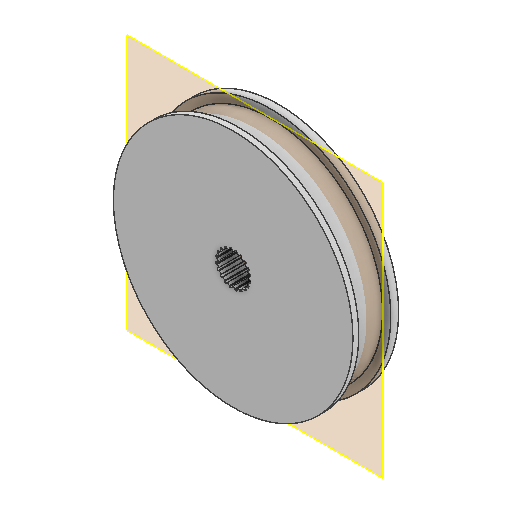
# Autodesk Inventor part: Diff Large Pulley
Saved by Autodesk Inventor 2025.2 (Build 292293000, 293)
## iProperties
Created: 2025-02-20
Part Number: Diff Large Pulley
Material: Generic
Document SubType Name: Modeling
Designer: Jakeg
Density: 1 g/cm^3
Appearance: Default
Author: Jakeg
Autodesk Inventor part; units mm, degrees
ref_plane "YZ Plane" through (0, 0, 0) normal (1, 0, 0) x (0, 1, 0)
ref_plane "XZ Plane" through (0, 0, 0) normal (0, 1, 0) x (-1, 0, 0)
ref_plane "XY Plane" through (0, 0, 0) normal (0, 0, 1) x (1, 0, 0)
sketch "Sketch1" plane through (0, 0, 0) normal (0, 0, 1) x (1, 0, 0)
  circle A0 centre (0, 0) radius 41.14
  dimension "d0" = 82.28
  constraints: 1 centre point, 1 coincident
  measures "d0" diameter of A0
extrude "Extrusion1" add sketch "Sketch1" along normal blind 15.7
ref_plane "Work Plane1" through (0, 0, 8.2) normal (0, 0, 1) x (1, 0, 0)
sketch "Sketch2" plane through (0, 0, 8.2) normal (0, 0, 1) x (1, 0, 0)
  circle A0 centre (0, 0) radius 38.3
  circle A1 centre (0, 0) radius 41.14
  dimension "d4" = 76.6
  constraints: 2 centre point, 2 coincident
  measures "d4" diameter of A0
extrude "Extrusion2" cut sketch "Sketch2" along normal mid plane 11
sketch "Sketch3" plane through (0, 0, 15.7) normal (0, 0, 1) x (1, 0, 0)
  circle A0 centre (0, 0) radius 6
  circle A1 centre (0, 20.32) radius 3.175
  circle A2 centre (0, -20.32) radius 3.175
  dimension "d7" = 12
  dimension "d13" = 6.35
  dimension "d14" = 20.32
  dimension "d15" = 6.35
  dimension "d16" = 20.32
  constraints: 3 centre point, 1 coincident
  measures "d7" diameter of A0
  measures "d13" diameter of A1
  measures "d14" distance of point (0, 0) A1.centre
  measures "d15" diameter of A2
  measures "d16" distance of point (0, 0) A2.centre
extrude "Extrusion3" cut sketch "Sketch3" against normal through all contours A0
sketch "Sketch5" plane through (0, 0, 15.7) normal (0, 0, 1) x (1, 0, 0)
  circle A0 centre (0, 0) radius 6 projected
  arc A1 (-1.2778, -5.5469) -> (-2.2267, -5.2386) centre (-1.8274, -5.6241) ccw
  arc A2 (-1.2783, -5.8289) -> (-1.2778, -5.5469) centre (-2.2681, -5.6859) ccw
  arc A3 (-1.2783, -5.8289) -> (-1.1583, -5.9977) centre (-1.1299, -5.8504) ccw
  arc A4 (-1.1583, -5.9977) -> (-0.7518, -6.0621) centre (0, 0) ccw
  arc A5 (-0.7518, -6.0621) -> (-0.5855, -5.9387) centre (-0.7333, -5.9132) ccw
  arc A6 (-0.4989, -5.6703) -> (-0.5855, -5.9387) centre (0.4, -6.1085) ccw
  arc A7 (0.4989, -5.6703) -> (-0.4989, -5.6703) centre (0, -5.9135) ccw
  arc A8 (0.5855, -5.9387) -> (0.4989, -5.6703) centre (-0.4, -6.1085) ccw
  arc A9 (0.5855, -5.9387) -> (0.7518, -6.0621) centre (0.7333, -5.9132) ccw
  arc A10 (0.7518, -6.0621) -> (1.1583, -5.9977) centre (0, 0) ccw
  arc A11 (1.1583, -5.9977) -> (1.2783, -5.8289) centre (1.1299, -5.8504) ccw
  arc A12 (1.2778, -5.5469) -> (1.2783, -5.8289) centre (2.2681, -5.6859) ccw
  arc A13 (2.2267, -5.2386) -> (1.2778, -5.5469) centre (1.8274, -5.6241) ccw
  arc A14 (2.392, -5.4671) -> (2.2267, -5.2386) centre (1.5072, -5.9331) ccw
  arc A15 (2.392, -5.4671) -> (2.5882, -5.5331) centre (2.5247, -5.3972) ccw
  arc A16 (2.5882, -5.5331) -> (2.955, -5.3462) centre (0, 0) ccw
  arc A17 (2.955, -5.3462) -> (3.017, -5.1486) centre (2.8824, -5.2149) ccw
  arc A18 (2.9293, -4.8806) -> (3.017, -5.1486) centre (3.9141, -4.7068) ccw
  arc A19 (3.7365, -4.2941) -> (2.9293, -4.8806) centre (3.4759, -4.7841) ccw
  arc A20 (3.9643, -4.4604) -> (3.7365, -4.2941) centre (3.2669, -5.177) ccw
  arc A21 (3.9643, -4.4604) -> (4.1714, -4.4624) centre (4.0689, -4.3529) ccw
  arc A22 (4.1714, -4.4624) -> (4.4624, -4.1714) centre (0, 0) ccw
  arc A23 (4.4624, -4.1714) -> (4.4604, -3.9643) centre (4.3529, -4.0689) ccw
  arc A24 (4.2941, -3.7365) -> (4.4604, -3.9643) centre (5.177, -3.2669) ccw
  arc A25 (4.8806, -2.9293) -> (4.2941, -3.7365) centre (4.7841, -3.4759) ccw
  arc A26 (5.1486, -3.017) -> (4.8806, -2.9293) centre (4.7068, -3.9141) ccw
  arc A27 (5.1486, -3.017) -> (5.3462, -2.955) centre (5.2149, -2.8824) ccw
  arc A28 (5.3462, -2.955) -> (5.5331, -2.5882) centre (0, 0) ccw
  arc A29 (5.5331, -2.5882) -> (5.4671, -2.392) centre (5.3972, -2.5247) ccw
  arc A30 (5.2386, -2.2267) -> (5.4671, -2.392) centre (5.9331, -1.5072) ccw
  arc A31 (5.5469, -1.2778) -> (5.2386, -2.2267) centre (5.6241, -1.8274) ccw
  arc A32 (5.8289, -1.2783) -> (5.5469, -1.2778) centre (5.6859, -2.2681) ccw
  arc A33 (5.8289, -1.2783) -> (5.9977, -1.1583) centre (5.8504, -1.1299) ccw
  arc A34 (5.9977, -1.1583) -> (6.0621, -0.7518) centre (0, 0) ccw
  arc A35 (6.0621, -0.7518) -> (5.9387, -0.5855) centre (5.9132, -0.7333) ccw
  arc A36 (5.6703, -0.4989) -> (5.9387, -0.5855) centre (6.1085, 0.4) ccw
  arc A37 (5.6703, 0.4989) -> (5.6703, -0.4989) centre (5.9135, 0) ccw
  arc A38 (5.9387, 0.5855) -> (5.6703, 0.4989) centre (6.1085, -0.4) ccw
  arc A39 (5.9387, 0.5855) -> (6.0621, 0.7518) centre (5.9132, 0.7333) ccw
  arc A40 (6.0621, 0.7518) -> (5.9977, 1.1583) centre (0, 0) ccw
  arc A41 (5.9977, 1.1583) -> (5.8289, 1.2783) centre (5.8504, 1.1299) ccw
  arc A42 (5.5469, 1.2778) -> (5.8289, 1.2783) centre (5.6859, 2.2681) ccw
  arc A43 (5.2386, 2.2267) -> (5.5469, 1.2778) centre (5.6241, 1.8274) ccw
  arc A44 (5.4671, 2.392) -> (5.2386, 2.2267) centre (5.9331, 1.5072) ccw
  arc A45 (5.4671, 2.392) -> (5.5331, 2.5882) centre (5.3972, 2.5247) ccw
  arc A46 (5.5331, 2.5882) -> (5.3462, 2.955) centre (0, 0) ccw
  arc A47 (5.3462, 2.955) -> (5.1486, 3.017) centre (5.2149, 2.8824) ccw
  arc A48 (4.8806, 2.9293) -> (5.1486, 3.017) centre (4.7068, 3.9141) ccw
  arc A49 (4.2941, 3.7365) -> (4.8806, 2.9293) centre (4.7841, 3.4759) ccw
  arc A50 (4.4604, 3.9643) -> (4.2941, 3.7365) centre (5.177, 3.2669) ccw
  arc A51 (4.4604, 3.9643) -> (4.4624, 4.1714) centre (4.3529, 4.0689) ccw
  arc A52 (4.4624, 4.1714) -> (4.1714, 4.4624) centre (0, 0) ccw
  arc A53 (4.1714, 4.4624) -> (3.9643, 4.4604) centre (4.0689, 4.3529) ccw
  arc A54 (3.7365, 4.2941) -> (3.9643, 4.4604) centre (3.2669, 5.177) ccw
  arc A55 (2.9293, 4.8806) -> (3.7365, 4.2941) centre (3.4759, 4.7841) ccw
  arc A56 (3.017, 5.1486) -> (2.9293, 4.8806) centre (3.9141, 4.7068) ccw
  arc A57 (3.017, 5.1486) -> (2.955, 5.3462) centre (2.8824, 5.2149) ccw
  arc A58 (2.955, 5.3462) -> (2.5882, 5.5331) centre (0, 0) ccw
  arc A59 (2.5882, 5.5331) -> (2.392, 5.4671) centre (2.5247, 5.3972) ccw
  arc A60 (2.2267, 5.2386) -> (2.392, 5.4671) centre (1.5072, 5.9331) ccw
  arc A61 (1.2778, 5.5469) -> (2.2267, 5.2386) centre (1.8274, 5.6241) ccw
  arc A62 (1.2783, 5.8289) -> (1.2778, 5.5469) centre (2.2681, 5.6859) ccw
  arc A63 (1.2783, 5.8289) -> (1.1583, 5.9977) centre (1.1299, 5.8504) ccw
  arc A64 (1.1583, 5.9977) -> (0.7518, 6.0621) centre (0, 0) ccw
  arc A65 (0.7518, 6.0621) -> (0.5855, 5.9387) centre (0.7333, 5.9132) ccw
  arc A66 (0.4989, 5.6703) -> (0.5855, 5.9387) centre (-0.4, 6.1085) ccw
  arc A67 (-0.4989, 5.6703) -> (0.4989, 5.6703) centre (0, 5.9135) ccw
  arc A68 (-0.5855, 5.9387) -> (-0.4989, 5.6703) centre (0.4, 6.1085) ccw
  arc A69 (-0.5855, 5.9387) -> (-0.7518, 6.0621) centre (-0.7333, 5.9132) ccw
  arc A70 (-0.7518, 6.0621) -> (-1.1583, 5.9977) centre (0, 0) ccw
  arc A71 (-1.1583, 5.9977) -> (-1.2783, 5.8289) centre (-1.1299, 5.8504) ccw
  arc A72 (-1.2778, 5.5469) -> (-1.2783, 5.8289) centre (-2.2681, 5.6859) ccw
  arc A73 (-2.2267, 5.2386) -> (-1.2778, 5.5469) centre (-1.8274, 5.6241) ccw
  arc A74 (-2.392, 5.4671) -> (-2.2267, 5.2386) centre (-1.5072, 5.9331) ccw
  arc A75 (-2.392, 5.4671) -> (-2.5882, 5.5331) centre (-2.5247, 5.3972) ccw
  arc A76 (-2.5882, 5.5331) -> (-2.955, 5.3462) centre (0, 0) ccw
  arc A77 (-2.955, 5.3462) -> (-3.017, 5.1486) centre (-2.8824, 5.2149) ccw
  arc A78 (-2.9293, 4.8806) -> (-3.017, 5.1486) centre (-3.9141, 4.7068) ccw
  arc A79 (-3.7365, 4.2941) -> (-2.9293, 4.8806) centre (-3.4759, 4.7841) ccw
  arc A80 (-3.9643, 4.4604) -> (-3.7365, 4.2941) centre (-3.2669, 5.177) ccw
  arc A81 (-3.9643, 4.4604) -> (-4.1714, 4.4624) centre (-4.0689, 4.3529) ccw
  arc A82 (-4.1714, 4.4624) -> (-4.4624, 4.1714) centre (0, 0) ccw
  arc A83 (-4.4624, 4.1714) -> (-4.4604, 3.9643) centre (-4.3529, 4.0689) ccw
  arc A84 (-4.2941, 3.7365) -> (-4.4604, 3.9643) centre (-5.177, 3.2669) ccw
  arc A85 (-4.8806, 2.9293) -> (-4.2941, 3.7365) centre (-4.7841, 3.4759) ccw
  arc A86 (-5.1486, 3.017) -> (-4.8806, 2.9293) centre (-4.7068, 3.9141) ccw
  arc A87 (-5.1486, 3.017) -> (-5.3462, 2.955) centre (-5.2149, 2.8824) ccw
  arc A88 (-5.3462, 2.955) -> (-5.5331, 2.5882) centre (0, 0) ccw
  arc A89 (-5.5331, 2.5882) -> (-5.4671, 2.392) centre (-5.3972, 2.5247) ccw
  arc A90 (-5.2386, 2.2267) -> (-5.4671, 2.392) centre (-5.9331, 1.5072) ccw
  arc A91 (-5.5469, 1.2778) -> (-5.2386, 2.2267) centre (-5.6241, 1.8274) ccw
  arc A92 (-5.8289, 1.2783) -> (-5.5469, 1.2778) centre (-5.6859, 2.2681) ccw
  arc A93 (-5.8289, 1.2783) -> (-5.9977, 1.1583) centre (-5.8504, 1.1299) ccw
  arc A94 (-5.9977, 1.1583) -> (-6.0621, 0.7518) centre (0, 0) ccw
  arc A95 (-6.0621, 0.7518) -> (-5.9387, 0.5855) centre (-5.9132, 0.7333) ccw
  arc A96 (-5.6703, 0.4989) -> (-5.9387, 0.5855) centre (-6.1085, -0.4) ccw
  arc A97 (-5.6703, -0.4989) -> (-5.6703, 0.4989) centre (-5.9135, 0) ccw
  arc A98 (-5.9387, -0.5855) -> (-5.6703, -0.4989) centre (-6.1085, 0.4) ccw
  arc A99 (-5.9387, -0.5855) -> (-6.0621, -0.7518) centre (-5.9132, -0.7333) ccw
  arc A100 (-6.0621, -0.7518) -> (-5.9977, -1.1583) centre (0, 0) ccw
  arc A101 (-5.9977, -1.1583) -> (-5.8289, -1.2783) centre (-5.8504, -1.1299) ccw
  arc A102 (-5.5469, -1.2778) -> (-5.8289, -1.2783) centre (-5.6859, -2.2681) ccw
  arc A103 (-5.2386, -2.2267) -> (-5.5469, -1.2778) centre (-5.6241, -1.8274) ccw
  arc A104 (-5.4671, -2.392) -> (-5.2386, -2.2267) centre (-5.9331, -1.5072) ccw
  arc A105 (-5.4671, -2.392) -> (-5.5331, -2.5882) centre (-5.3972, -2.5247) ccw
  arc A106 (-5.5331, -2.5882) -> (-5.3462, -2.955) centre (0, 0) ccw
  arc A107 (-5.3462, -2.955) -> (-5.1486, -3.017) centre (-5.2149, -2.8824) ccw
  arc A108 (-4.8806, -2.9293) -> (-5.1486, -3.017) centre (-4.7068, -3.9141) ccw
  arc A109 (-4.2941, -3.7365) -> (-4.8806, -2.9293) centre (-4.7841, -3.4759) ccw
  arc A110 (-4.4604, -3.9643) -> (-4.2941, -3.7365) centre (-5.177, -3.2669) ccw
  arc A111 (-4.4604, -3.9643) -> (-4.4624, -4.1714) centre (-4.3529, -4.0689) ccw
  arc A112 (-4.4624, -4.1714) -> (-4.1714, -4.4624) centre (0, 0) ccw
  arc A113 (-4.1714, -4.4624) -> (-3.9643, -4.4604) centre (-4.0689, -4.3529) ccw
  arc A114 (-3.7365, -4.2941) -> (-3.9643, -4.4604) centre (-3.2669, -5.177) ccw
  arc A115 (-2.9293, -4.8806) -> (-3.7365, -4.2941) centre (-3.4759, -4.7841) ccw
  arc A116 (-3.017, -5.1486) -> (-2.9293, -4.8806) centre (-3.9141, -4.7068) ccw
  arc A117 (-3.017, -5.1486) -> (-2.955, -5.3462) centre (-2.8824, -5.2149) ccw
  arc A118 (-2.955, -5.3462) -> (-2.5882, -5.5331) centre (0, 0) ccw
  arc A119 (-2.5882, -5.5331) -> (-2.392, -5.4671) centre (-2.5247, -5.3972) ccw
  arc A120 (-2.2267, -5.2386) -> (-2.392, -5.4671) centre (-1.5072, -5.9331) ccw
  point P0 (-3.9904, -4.4807)
  point P1 (-3.0283, -5.1797)
  point P2 (-5.1797, -3.0283)
  point P3 (-4.4807, -3.9904)
  point P4 (-5.862, -1.2794)
  point P5 (-5.4945, -2.4105)
  point P6 (-5.9705, 0.5947)
  point P7 (-5.9705, -0.5947)
  point P8 (-5.4945, 2.4105)
  point P9 (-5.862, 1.2794)
  point P10 (-4.4807, 3.9904)
  point P11 (-5.1797, 3.0283)
  point P12 (-3.0283, 5.1797)
  point P13 (-3.9904, 4.4807)
  point P14 (-1.2794, 5.862)
  point P15 (-2.4105, 5.4945)
  point P16 (0.5947, 5.9705)
  point P17 (-0.5947, 5.9705)
  point P18 (2.4105, 5.4945)
  point P19 (1.2794, 5.862)
  point P20 (3.9904, 4.4807)
  point P21 (3.0283, 5.1797)
  point P22 (5.1797, 3.0283)
  point P23 (4.4807, 3.9904)
  point P24 (5.862, 1.2794)
  point P25 (5.4945, 2.4105)
  point P26 (5.9705, -0.5947)
  point P27 (5.9705, 0.5947)
  point P28 (5.4945, -2.4105)
  point P29 (5.862, -1.2794)
  point P30 (4.4807, -3.9904)
  point P31 (5.1797, -3.0283)
  point P32 (3.0283, -5.1797)
  point P33 (3.9904, -4.4807)
  point P34 (1.2794, -5.862)
  point P35 (2.4105, -5.4945)
  point P36 (-0.5947, -5.9705)
  point P37 (0.5947, -5.9705)
  point P38 (-2.4105, -5.4945)
  point P39 (-1.2794, -5.862)
  dimension "d21" = 0
  dimension "d22" = 0
  constraints: 240 point on circle, 120 centre point, 1 coincident, 1 other
  measures "d21" distance of point (0, 0) A4.centre
  measures "d22" distance of A4.centre point (0, 0)
extrude "Extrusion5" add sketch "Sketch5" against normal blind 15.7 contours A0 A35 A36 A37 A38 A39 | A0 A41 A40 A39 | A35 A34 A33 A0 | A41 A42 A43 A44 A45 A0 | A0 A29 A30 A31 A32 A33 | A0 A47 A46 A45 | A29 A28 A27 A0 | A47 A48 A49 A50 A51 A0 | A0 A23 A24 A25 A26 A27 | A0 A53 A52 A51 | A23 A22 A21 A0 | A53 A54 A55 A56 A57 A0 | A0 A17 A18 A19 A20 A21 | A0 A59 A58 A57 | A17 A16 A15 A0 | A59 A60 A61 A62 A63 A0 | A0 A11 A12 A13 A14 A15 | A0 A65 A64 A63 | A11 A10 A9 A0 | A65 A66 A67 A68 A69 A0 | A0 A5 A6 A7 A8 A9 | A0 A71 A70 A69 | A5 A4 A3 A0 | A71 A72 A73 A74 A75 A0 | A0 A119 A120 A1 A2 A3 | A0 A77 A76 A75 | A119 A118 A117 A0 | A77 A78 A79 A80 A81 A0 | A0 A113 A114 A115 A116 A117 | A0 A83 A82 A81 | A113 A112 A111 A0 | A83 A84 A85 A86 A87 A0 | A0 A107 A108 A109 A110 A111 | A0 A89 A88 A87 | A107 A106 A105 A0 | A89 A90 A91 A92 A93 A0 | A0 A101 A102 A103 A104 A105 | A0 A95 A94 A93 | A101 A100 A99 A0 | A95 A96 A97 A98 A99 A0
body "Solid1"
